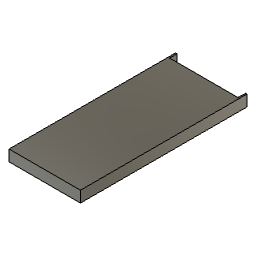
pils case (Autodesk Fusion 360 design; units mm, degrees)
Autodesk Fusion 360 part; units mm, degrees
sketch "Sketch1" plane through (0, 0, 0) normal (0, 0, 1) x (1, 0, 0)
  line L0 (0, 0) -> (48, 0)
  line L1 (48, 0) -> (48, 112)
  line L2 (48, 112) -> (0, 112)
  line L3 (0, 112) -> (0, 0)
  line L4 (1, 1) -> (47, 1)
  line L5 (47, 1) -> (47, 111)
  line L6 (47, 111) -> (1, 111)
  line L7 (1, 111) -> (1, 1)
  dimension "d1" = 48
  dimension "d2" = 112
  constraint horizontal L0
  constraint vertical L1
  constraint horizontal L2
  constraint vertical L3
  constraint coincident L0.start L3.end
  constraint horizontal L4
  constraint vertical L5
  constraint horizontal L6
  constraint vertical L7
  measures "d1" distance of L0.start L0.end
  measures "d2" distance of L0.start L2.end
extrude "Extrude1" add sketch "Sketch1" along normal blind 5.5
extrude "Extrude2" add sketch "Sketch1" against normal blind 1 contours L0 L1 L2 L3 | L4 L5 L6 L7
sketch "Sketch2" plane through (0, 0, 5.5) normal (0, 0, 1) x (-1, 0, 0)
  line L0 (-1, -1) -> (-1, -111)
  line L1 (-1, -111) -> (-47, -111)
  line L2 (-47, -111) -> (-47, -1)
  line L3 (-47, -1) -> (-1, -1)
  line L4 (0, -112) -> (0, 0)
  line L5 (0, 0) -> (-48, 0)
  line L6 (-48, 0) -> (-48, -112)
  line L7 (-48, -112) -> (0, -112)
  line L8 (-48, 0) -> (0, 0)
  line L9 (0, 0) -> (0, -112)
  line L10 (0, -112) -> (-48, -112)
  line L11 (-48, -112) -> (-48, 0)
  constraint horizontal L8
  constraint vertical L9
  constraint horizontal L10
  constraint vertical L11
  constraint coincident L4.start L7.end
  constraint coincident L5.end L6.start
extrude "Extrude3" add sketch "Sketch2" along normal blind 1 contours L0 L1 L2 L3 | L4 L5 L6 L7 L8 L9 L10 L11
sketch "Sketch3" plane through (0, 112, 0) normal (0, 1, 0) x (-1, 0, 0)
  line L0 (0, -1) -> (0, 6.5)
  line L1 (0, 6.5) -> (-48, 6.5)
  line L2 (-48, 6.5) -> (-48, -1)
  line L3 (-48, -1) -> (0, -1)
  line L4 (-47, 1) -> (-1, 1)
  line L5 (-1, 1) -> (-1, 6.5)
  line L6 (-1, 6.5) -> (-47, 6.5)
  line L7 (-47, 6.5) -> (-47, 1)
  dimension "d9" = 46
  constraint horizontal L4
  constraint vertical L5
  constraint horizontal L6
  constraint vertical L7
  measures "d9" distance of L4.start L4.end
extrude "Extrude4" cut sketch "Sketch3" against normal blind 5 contours L1 L4 L5 L6 L7
fillet "Fillet1" radius 2 1 edges at (24, 111, 0)
